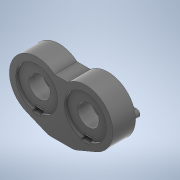
# Autodesk Inventor part: switch_mount_2
Saved by Autodesk Inventor 2022.2 (Build 262287000, 287)
## iProperties
Created: 2022-01-27
Part Number: switch_mount_2
Material: Generic
Document SubType Name: Modeling
Designer: hugof
Density: 1 g/cm^3
Appearance: Default
Author: hugof
Autodesk Inventor part; units mm, degrees
ref_plane "YZ Plane" through (0, 0, 0) normal (1, 0, 0) x (0, 1, 0)
ref_plane "XZ Plane" through (0, 0, 0) normal (0, 1, 0) x (-1, 0, 0)
ref_plane "XY Plane" through (0, 0, 0) normal (0, 0, 1) x (1, 0, 0)
sketch "Sketch2" plane through (0, 0, 0) normal (0, 0, 1) x (1, 0, 0)
  circle A0 centre (0, 0) radius 5.95
  line L0 (0, 0) -> (-4.55, 0)
  line L1 (0, 0) -> (4.55, 0)
  line L2 (0, 0) -> (0, 4.55)
  line L3 (0, 0) -> (0, -4.55)
  line L4 (-4.55, 0) -> (-4.55, -1.8847)
  line L5 (0, 0) -> (2.5958, -2.5958)
  line L6 (0, 0) -> (3.671, 0) construction
  line L7 (3.2173, -3.2173) -> (-3.2173, 3.2173)
  line L8 (0, 0) -> (-3.2173, -3.2173)
  line L9 (0, 0) -> (3.2173, 3.2173)
  line L10 (-3.2173, -3.2173) -> (-1.8847, -4.55)
  line L11 (-3.2173, -3.2173) -> (-4.55, -1.8847)
  line L12 (3.2173, -3.2173) -> (1.8847, -4.55)
  line L13 (3.2173, -3.2173) -> (4.55, -1.8847)
  line L14 (4.55, 0) -> (4.55, -1.8847)
  line L15 (4.55, 0) -> (4.55, 1.8847)
  line L16 (3.2173, 3.2173) -> (4.55, 1.8847)
  line L17 (3.2173, 3.2173) -> (1.8847, 4.55)
  line L18 (0, 4.55) -> (1.8847, 4.55)
  line L19 (0, 4.55) -> (-1.8847, 4.55)
  line L20 (-3.2173, 3.2173) -> (-1.8847, 4.55)
  line L21 (-3.2173, 3.2173) -> (-4.55, 1.8847)
  line L22 (0, -4.55) -> (1.8847, -4.55)
  line L23 (0, -4.55) -> (-1.8847, -4.55)
  line L24 (-4.55, 0) -> (-4.55, 1.8847)
  line L25 (5.95, 0) -> (7.95, 0)
  circle A1 centre (13.9, 0) radius 5.95
  line L26 (6.95, 0) -> (6.95, 2.7112)
  line L27 (-7.95, 7.8017) -> (21.85, 7.8017)
  line L28 (18.45, 0) -> (18.45, 1.8847)
  line L29 (18.45, 0) -> (18.45, -1.8847)
  line L30 (13.9, 0) -> (18.45, 0)
  line L31 (13.9, 0) -> (13.9, 4.55)
  line L32 (13.9, 0) -> (13.9, -4.55)
  line L33 (13.9, -4.55) -> (15.7847, -4.55)
  line L34 (13.9, 4.55) -> (12.0153, 4.55)
  line L35 (13.9, 0) -> (10.6827, 3.2173)
  line L36 (13.9, 0) -> (11.3042, -2.5958)
  line L37 (13.9, -4.55) -> (12.0153, -4.55)
  line L38 (10.6827, 3.2173) -> (9.35, 1.8847)
  line L39 (9.35, 0) -> (9.35, -1.8847)
  line L40 (10.6827, -3.2173) -> (17.1173, 3.2173)
  line L41 (10.6827, -3.2173) -> (9.35, -1.8847)
  circle A2 centre (13.9, 0) radius 5.95
  line L42 (10.6827, -3.2173) -> (12.0153, -4.55)
  line L43 (13.9, 0) -> (9.35, 0)
  line L44 (9.35, 0) -> (9.35, 1.8847)
  line L45 (13.9, 0) -> (10.229, 0) construction
  line L46 (17.1173, 3.2173) -> (15.7847, 4.55)
  line L47 (10.6827, 3.2173) -> (12.0153, 4.55)
  line L48 (13.9, 4.55) -> (15.7847, 4.55)
  line L49 (17.1173, 3.2173) -> (18.45, 1.8847)
  line L50 (17.1173, -3.2173) -> (18.45, -1.8847)
  line L51 (17.1173, -3.2173) -> (15.7847, -4.55)
  line L52 (13.9, 0) -> (17.1173, -3.2173)
  line L53 (21.85, 7.8017) -> (21.85, -7.8017)
  line L54 (-7.95, 7.8017) -> (-7.95, -7.8017)
  line L55 (21.85, -7.8017) -> (-7.95, -7.8017)
  dimension "d0" = 4.55
  dimension "d1" = 4.55
  dimension "d2" = 4.55
  dimension "d3" = 4.55
  dimension "d4" = 45
  constraints: 112 end point, 20 symmetric about line, 9 perpendicular, 7 horizontal, 7 vertical, 3 horizontal alignment, 3 midpoint, 2 coincident, 1 equal length, 6 other
  measures "d0" distance of L0.start L0.end
  measures "d1" distance of L0.start L1.end
  measures "d2" distance of L0.start L2.end
  measures "d3" distance of L0.start L3.end
  measures "d4" angle of L5 L6
extrude "Extrusion1" add sketch "Sketch2" along normal blind 1.6 contours A0 | A1 | L27 L53 L55 L54
sketch "Sketch3" plane through (0, 0, 1.6) normal (0, 0, 1) x (1, 0, 0)
  circle A0 centre (0, 0) radius 3.05
  line L0 (21.85, 7.8017) -> (-7.95, 7.8017) projected
  line L1 (-7.95, 7.8017) -> (-7.95, -7.8017) projected
  line L2 (-4.55, 1.8847) -> (-1.8847, 4.55) projected
  line L3 (-1.8847, 4.55) -> (1.8847, 4.55) projected
  line L4 (1.8847, 4.55) -> (4.55, 1.8847) projected
  line L5 (4.55, 1.8847) -> (4.55, -1.8847) projected
  line L6 (4.55, -1.8847) -> (1.8847, -4.55) projected
  line L7 (1.8847, -4.55) -> (-1.8847, -4.55) projected
  line L8 (-1.8847, -4.55) -> (-4.55, -1.8847) projected
  line L9 (-4.55, -1.8847) -> (-4.55, 1.8847) projected
  line L10 (18.45, -1.8847) -> (15.7847, -4.55) projected
  line L11 (15.7847, -4.55) -> (12.0153, -4.55) projected
  line L12 (12.0153, -4.55) -> (9.35, -1.8847) projected
  line L13 (9.35, -1.8847) -> (9.35, 1.8847) projected
  line L14 (9.35, 1.8847) -> (12.0153, 4.55) projected
  line L15 (12.0153, 4.55) -> (15.7847, 4.55) projected
  line L16 (15.7847, 4.55) -> (18.45, 1.8847) projected
  line L17 (18.45, 1.8847) -> (18.45, -1.8847) projected
  circle A1 centre (13.9, 0) radius 3.05
  line L18 (9.35, -1.8847) -> (9.35, 1.8847) projected
  line L19 (9.35, 0) -> (10.85, 0)
  line L20 (18.45, 1.8847) -> (18.45, -1.8847) projected
  line L21 (18.45, 0) -> (16.95, 0)
  line L22 (3.05, 0) -> (4.55, 0)
  line L23 (4.55, 1.8847) -> (4.55, -1.8847) projected
  line L24 (-4.55, -1.8847) -> (-4.55, 1.8847) projected
  line L25 (-4.55, 0) -> (-3.05, 0)
  line L26 (13.9, 0) -> (21.85, 0)
  line L27 (21.85, 0) -> (21.85, 7.95)
  line L28 (21.85, 0) -> (21.85, -7.8017)
  line L29 (-7.95, -7.8017) -> (21.85, -7.8017) projected
  line L30 (21.85, -7.8017) -> (21.85, 7.8017) projected
  dimension "d7" = 6.1
  dimension "d8" = 6.1
  constraints: 14 end point, 4 midpoint, 4 point on circle, 2 centre point, 2 point on line, 1 coincident, 1 horizontal, 1 perpendicular, 1 vertical
  measures "d7" diameter of A0
  measures "d8" diameter of A1
extrude "Extrusion2" add sketch "Sketch3" along normal blind 4 contours L22 L5 L6 L7 L8 L9 L25 A0 | A0 L25 L9 L2 L3 L4 L5 L22 | L27 L28 L29 L1 L0 | L10 L11 L12 L13 L19 A1 L21 L17 | L21 A1 L19 L13 L14 L15 L16 L17
sketch "Sketch4" plane through (0, 0, 5.6) normal (0, 0, 1) x (1, 0, 0)
  line L0 (21.85, 7.8017) -> (21.85, -7.8017)
  line L1 (21.85, -7.8017) -> (-8.35, -7.8017)
  line L2 (-7.95, -7.8017) -> (21.85, -7.8017)
  line L3 (-7.95, 7.8017) -> (-7.95, -7.8017)
  circle A0 centre (0, 0) radius 5.95
  circle A1 centre (13.9, 0) radius 5.95
  line L4 (21.85, 7.8017) -> (-7.95, 7.8017)
  line L5 (13.9, 0) -> (13.9, 7.8017)
  line L6 (13.9, 0) -> (13.9, -7.8017)
  line L7 (0, 0) -> (0, -7.8017)
  line L8 (0, 0) -> (0, 7.8017)
  line L9 (13.9, -5.95) -> (13.9, -6.35)
  line L10 (13.9, -6.35) -> (15, -6.35)
  line L11 (13.9, -6.35) -> (12.8, -6.35)
  line L12 (15, -6.35) -> (15, -5.8474)
  line L13 (12.8, -6.35) -> (12.8, -5.8474)
  line L14 (0, -5.95) -> (0, -6.35)
  line L15 (0, -6.35) -> (1.1, -6.35)
  line L16 (0, -6.35) -> (-1.1, -6.35)
  line L17 (1.1, -6.35) -> (1.1, -5.8474)
  line L18 (-1.1, -6.35) -> (-1.1, -5.8474)
  point P0 (0, 0)
  point P1 (-7.95, 0)
  point P2 (-59.6, 0)
  dimension "d28" = 0.4
  dimension "d29" = 1.1
  dimension "d30" = 1.1
  dimension "d31" = 0.4
  dimension "d32" = 1.1
  dimension "d33" = 1.1
  constraints: 38 end point, 6 point on line, 5 horizontal, 2 centre point, 2 vertical, 1 perpendicular
  measures "d28" distance of L9.start L10.start
  measures "d29" distance of L10.start L12.start
  measures "d30" distance of L10.start L11.end
  measures "d31" distance of L14.start L15.start
  measures "d32" distance of L15.start L17.start
  measures "d33" distance of L15.start L16.end
extrude "Extrusion4" add sketch "Sketch4" along normal blind 0.8 contours L0 L1 L6 L10 L12 A1 L5 L4 | L5 A1 L13 L11 L6 L1 L7 L15 L17 A0 L8 L4 | L8 A0 L18 L16 L7 L1 L3 L4
extrude "Extrusion5" cut sketch "Sketch4" against normal blind 0.8 contours L11 L13 A1 L6 | L6 A1 L12 L10 | L16 L18 A0 L7 | L7 A0 L17 L15
fillet "Fillet3" radius 1 2 edges at (13.9, -5.95, 5.6) (0, -5.95, 5.6)
sketch "Sketch5" plane through (0, 0, 6.4) normal (0, 0, 1) x (1, 0, 0)
  arc A0 (15, -5.8474) -> (12.8, -5.8474) centre (13.9, 0) ccw projected
  arc A1 (1.1, -5.8474) -> (-1.1, -5.8474) centre (0, 0) ccw projected
  circle A2 centre (0, 0) radius 7.8017
  circle A3 centre (13.9, 0) radius 7.8017
  line L0 (0, 7.8017) -> (13.9, 7.8017)
  line L1 (13.9, -7.8017) -> (0, -7.8017)
  line L2 (21.85, 7.8017) -> (-7.95, 7.8017) projected
  line L3 (0, 7.8017) -> (-7.95, 7.8017)
  line L4 (-7.95, 7.8017) -> (-7.95, -7.8017) projected
  line L5 (-7.95, 7.8017) -> (-7.95, -7.8017)
  line L6 (-7.95, -7.8017) -> (0, -7.8017)
  line L7 (5.0462, 5.95) -> (8.8538, 5.95)
  line L8 (18.9462, 5.95) -> (21.85, 5.95)
  line L9 (21.85, -6.2271) -> (18.6, -6.2271)
  line L10 (9.2, -6.2271) -> (4.7, -6.2271)
  line L11 (13.9, 7.8017) -> (21.85, 7.8017)
  line L12 (-7.95, -7.8017) -> (21.85, -7.8017) projected
  line L13 (21.85, -7.8017) -> (21.85, 7.8017) projected
  line L14 (21.85, -7.8017) -> (21.85, 7.8017)
  line L15 (21.85, -7.8017) -> (13.9, -7.8017)
  line L16 (21.85, 7.8017) -> (-7.95, 7.8017)
  line L17 (-7.95, -7.8017) -> (21.85, -7.8017)
  line L18 (4.7, -6.2271) -> (9.2, -6.2271)
  line L19 (5.0462, 5.95) -> (8.8538, 5.95)
  line L20 (21.85, -7.8017) -> (13.9, -7.8017)
  line L21 (0, -7.8017) -> (13.9, -7.8017)
  line L22 (0, -7.8017) -> (-7.95, -7.8017)
  line L23 (-7.95, 7.8017) -> (-7.95, -7.8017) projected
  line L24 (-7.95, -7.8017) -> (-7.95, 7.8017)
  line L25 (-7.95, 7.8017) -> (0, 7.8017)
  line L26 (13.9, 7.8017) -> (0, 7.8017)
  line L27 (21.85, 7.8017) -> (13.9, 7.8017)
  line L28 (21.85, 7.8017) -> (21.85, -7.8017)
  line L29 (-7.95, 7.8017) -> (21.85, 7.8017)
  line L30 (21.85, -7.8017) -> (-7.95, -7.8017)
  line L31 (-7.95, -7.8017) -> (-7.95, 7.8017)
  point P0 (0, 0)
  point P1 (-5.45, 7.8017)
  point P2 (-5.45, -7.8017)
  point P3 (49.15, -7.8017)
  point P4 (6.95, 3.5446)
  point P5 (6.95, -3.5446)
  constraints: 54 end point, 10 point on circle, 9 tangent, 7 collinear, 5 point on line, 4 perpendicular, 2 centre point, 2 coincident, 2 horizontal, 2 parallel, 1 vertical
extrude "Extrusion6" cut sketch "Sketch5" against normal through all contours A2 L0 A3 L7 | A2 L6 L4 L2 | A2 L10 A3 L1 | L2 L13 L8 A3 | A3 L9 L13 L12 | L8 L13 L9 A3
sketch "Sketch7" plane through (0, 0, 6.4) normal (0, 0, 1) x (1, 0, 0)
  arc A0 (9.2, -6.2271) -> (8.8538, 5.95) centre (13.9, 0) ccw projected
  line L0 (8.8538, 5.95) -> (5.0462, 5.95) projected
  arc A1 (5.0462, 5.95) -> (4.7, -6.2271) centre (0, 0) ccw projected
  line L1 (4.7, -6.2271) -> (9.2, -6.2271) projected
  line L2 (15, -6.35) -> (12.8, -6.35) projected
  line L3 (12.8, -6.35) -> (12.8, -5.8474) projected
  arc A2 (15, -5.8474) -> (12.8, -5.8474) centre (13.9, 0) ccw projected
  line L4 (15, -5.8474) -> (15, -6.35) projected
  arc A3 (1.1, -5.8474) -> (-1.1, -5.8474) centre (0, 0) ccw projected
  line L5 (1.1, -5.8474) -> (1.1, -6.35) projected
  line L6 (1.1, -6.35) -> (-1.1, -6.35) projected
  line L7 (-1.1, -6.35) -> (-1.1, -5.8474) projected
  arc A4 (5.0462, 5.95) -> (4.7, -6.2271) centre (0, 0) ccw projected
  arc A5 (9.2, -6.2271) -> (8.8538, 5.95) centre (13.9, 0) ccw projected
  line L8 (7.0416, -9.3601) -> (7.0416, -11.3601)
  line L9 (0, -7.8017) -> (7.0416, -11.3601)
  line L10 (13.9, -7.8017) -> (7.0416, -11.3601)
  line L11 (4.7, -6.2271) -> (6.973, -3.9772)
  line L12 (9.2, -6.2271) -> (4.7, -6.2271) projected
  line L13 (6.973, -3.9772) -> (9.2, -6.2271)
  line L14 (4.7, -6.2271) -> (6.973, 0)
  line L15 (6.973, 0) -> (9.2, -6.2271)
  line L16 (4.7, -6.2271) -> (9.2, -6.2271) projected
  line L17 (13.9, -7.8017) -> (9.2, -6.2271)
  line L18 (4.7, -6.2271) -> (0, -7.8017)
  arc A6 (5.0462, 5.95) -> (4.7, -6.2271) centre (0, 0) ccw projected
  line L19 (7.0416, -11.3601) -> (16.932, -7.1885)
  line L20 (7.0416, -11.3601) -> (-2.9849, -7.2082)
  point P0 (0, 0)
  dimension "d49" = 2
  constraints: 22 end point, 4 point on circle, 2 tangent, 1 perpendicular, 1 vertical
  measures "d49" distance of L8.start L8.end
extrude "Extrusion8" add sketch "Sketch7" against normal up to surface (6.4 mm away) contours A0 L10 L9 A1 L1 | A0 L19 L10 | L20 A1 L9
chamfer "Chamfer4" distance 4 angle 45 1 edges at (7.0416, -11.3601, 3.2)
fillet "Fillet7" radius 4 2 edges at (10.7272, -9.8056, 3.2) (3.346, -9.8297, 3.2)
sketch "Sketch10" plane through (0, 0, 0) normal (0, 0, -1) x (-1, 0, 0)
  line L0 (-16.932, -7.1885) -> (-11.4664, -9.4938) projected
  line L1 (-4.1482, -9.8271) -> (-9.925, -9.8082) projected
  arc A0 (-11.4664, -9.4938) -> (-9.925, -9.8082) centre (-9.9119, -5.8082) ccw projected
  arc A1 (-4.1482, -9.8271) -> (-2.6048, -9.5228) centre (-4.1351, -5.8271) ccw projected
  line L2 (-16.932, -7.1885) -> (-11.4664, -9.4938)
  line L3 (-4.1482, -9.8271) -> (-9.925, -9.8082)
  arc A2 (-11.4664, -9.4938) -> (-9.925, -9.8082) centre (-9.9119, -5.8082) ccw
  arc A3 (-4.1482, -9.8271) -> (-2.6048, -9.5228) centre (-4.1351, -5.8271) ccw
  arc A4 (-12.8, -5.8474) -> (-15, -5.8474) centre (-13.9, 0) ccw projected
  line L4 (-18.45, -1.8847) -> (-15.7847, -4.55) projected
  line L5 (-18.45, 1.8847) -> (-18.45, -1.8847) projected
  line L6 (-15.7847, 4.55) -> (-18.45, 1.8847) projected
  line L7 (-12.0153, 4.55) -> (-15.7847, 4.55) projected
  line L8 (-9.35, 1.8847) -> (-12.0153, 4.55) projected
  line L9 (-9.35, -1.8847) -> (-9.35, 1.8847) projected
  line L10 (-12.0153, -4.55) -> (-9.35, -1.8847) projected
  line L11 (-15.7847, -4.55) -> (-12.0153, -4.55) projected
  line L12 (4.55, 1.8847) -> (1.8847, 4.55) projected
  line L13 (4.55, -1.8847) -> (4.55, 1.8847) projected
  line L14 (1.8847, -4.55) -> (4.55, -1.8847) projected
  line L15 (-1.8847, -4.55) -> (1.8847, -4.55) projected
  line L16 (-4.55, -1.8847) -> (-1.8847, -4.55) projected
  line L17 (-4.55, 1.8847) -> (-4.55, -1.8847) projected
  line L18 (-1.8847, 4.55) -> (-4.55, 1.8847) projected
  line L19 (1.8847, 4.55) -> (-1.8847, 4.55) projected
  arc A5 (-4.1482, -9.8271) -> (-2.6048, -9.5228) centre (-4.1351, -5.8271) ccw projected
  line L20 (-2.6048, -9.5228) -> (2.9849, -7.2082) projected
  arc A6 (2.9849, -7.2082) -> (-5.0462, 5.95) centre (0, 0) ccw projected
  line L21 (-5.0462, 5.95) -> (-8.8538, 5.95) projected
  arc A7 (-8.8538, 5.95) -> (-16.932, -7.1885) centre (-13.9, 0) ccw projected
  line L22 (-16.932, -7.1885) -> (-11.4664, -9.4938) projected
  arc A8 (-11.4664, -9.4938) -> (-9.925, -9.8082) centre (-9.9119, -5.8082) ccw projected
  line L23 (-4.1482, -9.8271) -> (-9.925, -9.8082) projected
  arc A9 (-15, -5.8474) -> (-12.8, -5.8474) centre (-13.9, 0) ccw projected
  circle A10 centre (0, 0) radius 3.05 projected
  line L24 (4.55, -1.8847) -> (4.55, 1.8847) projected
  line L25 (4.55, 1.8847) -> (1.8847, 4.55) projected
  line L26 (1.8847, 4.55) -> (-1.8847, 4.55) projected
  line L27 (-1.8847, 4.55) -> (-4.55, 1.8847) projected
  line L28 (-4.55, 1.8847) -> (-4.55, -1.8847) projected
  line L29 (-4.55, -1.8847) -> (-1.8847, -4.55) projected
  line L30 (-1.8847, -4.55) -> (1.8847, -4.55) projected
  line L31 (1.8847, -4.55) -> (4.55, -1.8847) projected
  circle A11 centre (-13.9, 0) radius 3.05 projected
  line L32 (-18.45, 1.8847) -> (-18.45, -1.8847) projected
  line L33 (-18.45, -1.8847) -> (-15.7847, -4.55) projected
  line L34 (-15.7847, -4.55) -> (-12.0153, -4.55) projected
  line L35 (-12.0153, -4.55) -> (-9.35, -1.8847) projected
  line L36 (-9.35, -1.8847) -> (-9.35, 1.8847) projected
  line L37 (-9.35, 1.8847) -> (-12.0153, 4.55) projected
  line L38 (-12.0153, 4.55) -> (-15.7847, 4.55) projected
  line L39 (-15.7847, 4.55) -> (-18.45, 1.8847) projected
  arc A12 (1.1, -5.8474) -> (-1.1, -5.8474) centre (0, 0) ccw projected
  arc A13 (-1.1, -5.8474) -> (1.1, -5.8474) centre (0, 0) ccw projected
  line L40 (-16.932, -7.1885) -> (3.032, -7.1885)
  line L41 (3.032, -7.1885) -> (-2.6048, -9.5228)
  line L42 (-9.925, -9.8082) -> (-4.1482, -9.8271) projected
  arc A14 (2.9849, -7.2082) -> (-5.0462, 5.95) centre (0, 0) ccw projected
  line L43 (-7.0366, -7.1885) -> (-7.0366, -9.8176)
  line L44 (-7.0366, -11.3581) -> (-11.3581, -11.3581)
  line L45 (-7.0366, -11.3581) -> (-2.6048, -11.3581)
  line L46 (3.032, -7.1885) -> (-2.6048, -11.3581)
  line L47 (-16.932, -7.1885) -> (-11.3581, -11.3581)
  point P0 (-2.6048, -9.5228)
  constraints: 18 end point, 5 point on circle, 4 point on line, 3 horizontal, 2 centre point, 1 concentric, 1 midpoint
extrude "Extrusion10" add sketch "Sketch10" along normal blind 10 contours L40 L43 L1 A0 L0 | L40 A6 L20 A1 L1 L43
sketch "Sketch12" plane through (-3.032, -7.1885, 0) normal (0, 1, 0) x (1, 0, 0)
  line L0 (19.964, 0) -> (0, 0) projected
  line L1 (19.964, 0) -> (19.964, 10) projected
  line L2 (0, 10) -> (19.964, 10) projected
  line L3 (0, 0) -> (0, 10) projected
  line L4 (0, 10) -> (19.964, 10) projected
  line L5 (19.964, 10) -> (0, 0)
  line L6 (0, 10) -> (19.964, 0)
  circle A0 centre (9.982, 5) radius 1.5
  circle A1 centre (9.982, 5) radius 2.9
  point P0 (3.032, 0)
  dimension "d75" = 3
  dimension "d82" = 5.8
  constraints: 4 end point, 2 centre point, 1 coincident, 1 midpoint
  measures "d75" diameter of A0
  measures "d82" diameter of A1
fillet "Fillet8" radius 1 2 edges at (16.932, -7.1885, -5) (-3.032, -7.1885, -5)
extrude "Extrusion12" cut sketch "Sketch12" along normal through all both and the other way through all contours A0 L5 L6 | L6 L5 A0 | A0 L6 L5 | L5 L6 A0
sketch "Sketch14" plane through (4.1482, -9.8271, -10) normal (0.003274, -0.9999946, 0) x (0.9999946, 0.003274, 0)
  ellipse E0 centre (2.8018, 5) end of major axis (4.3018, 5) minor radius 1.5 projected
  circle A0 centre (2.8018, 5) radius 2.7
  point P0 (-4.116, 10)
  dimension "d81" = 5.4
  constraints: 1 centre point, 1 coincident
  measures "d81" diameter of A0
extrude "Extrusion14" cut sketch "Sketch12" against normal blind 1 contours A1 L5 A0 L6 | L6 A0 L5 A1 | A1 L6 A0 L5 | L5 A0 L6 A1 | A0 L5 L6 | L6 L5 A0 | A0 L6 L5 | L5 L6 A0
body "Solid1"
